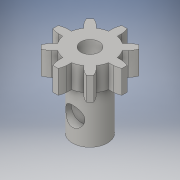
# Autodesk Inventor part: Small Gear
Saved by Autodesk Inventor 2016 (Build 200138000, 138)
## iProperties
Created: 2016-04-12
Part Number: Small Gear
Material: Generic
Document SubType Name: Modeling
Designer: rmarkowi
Density: 1 g/cm^3
Appearance: Default
Author: rmarkowi
Autodesk Inventor part; units mm, degrees
ref_plane "YZ Plane" through (0, 0, 0) normal (1, 0, 0) x (0, 1, 0)
sketch "Sketch1" plane through (0, 0, 0) normal (0, 1, 0) x (-1, 0, 0)
  line L0 (-7.4806, -1.1906) -> (-6.2374, -1.1906)
  arc A0 (-9.4068, -0.7091) -> (-7.4806, -1.1906) centre (-6.9988, 4.8297) ccw
  line L1 (-9.4068, 0) -> (-9.4068, -0.7091)
  line L2 (-9.4068, 0) -> (-9.4068, 0.7091)
  line L3 (-7.4806, 1.1906) -> (-6.2374, 1.1906)
  arc A1 (-7.4806, 1.1906) -> (-9.4068, 0.7091) centre (-6.9988, -4.8297) ccw
  line L4 (-7.4806, -1.1906) -> (-6.2374, -1.1906)
  arc A2 (-9.4068, -0.7091) -> (-7.4806, -1.1906) centre (-6.9988, 4.8297) ccw
  line L5 (-9.4068, 0) -> (-9.4068, -0.7091)
  line L6 (-9.4068, 0) -> (-9.4068, 0.7091)
  line L7 (-7.4806, 1.1906) -> (-6.2374, 1.1906)
  arc A3 (-7.4806, 1.1906) -> (-9.4068, 0.7091) centre (-6.9988, -4.8297) ccw
  line L8 (-4.4477, -6.1315) -> (-3.5686, -5.2524)
  line L9 (-4.4477, -6.1315) -> (-3.5686, -5.2524)
  line L10 (-6.6516, -6.6516) -> (-6.1502, -7.153)
  line L11 (-6.6516, -6.6516) -> (-6.1502, -7.153)
  line L12 (-6.6516, -6.6516) -> (-7.153, -6.1502)
  line L13 (-6.6516, -6.6516) -> (-7.153, -6.1502)
  line L14 (-6.1315, -4.4477) -> (-5.2524, -3.5686)
  line L15 (-6.1315, -4.4477) -> (-5.2524, -3.5686)
  arc A4 (-6.1315, -4.4477) -> (-7.153, -6.1502) centre (-1.5338, -8.364) ccw
  arc A5 (-6.1315, -4.4477) -> (-7.153, -6.1502) centre (-1.5338, -8.364) ccw
  arc A6 (-6.1502, -7.153) -> (-4.4477, -6.1315) centre (-8.364, -1.5338) ccw
  arc A7 (-6.1502, -7.153) -> (-4.4477, -6.1315) centre (-8.364, -1.5338) ccw
  line L16 (1.1906, -7.4806) -> (1.1906, -6.2374)
  line L17 (1.1906, -7.4806) -> (1.1906, -6.2374)
  line L18 (0, -9.4068) -> (0.7091, -9.4068)
  line L19 (0, -9.4068) -> (0.7091, -9.4068)
  line L20 (0, -9.4068) -> (-0.7091, -9.4068)
  line L21 (0, -9.4068) -> (-0.7091, -9.4068)
  line L22 (-1.1906, -7.4806) -> (-1.1906, -6.2374)
  line L23 (-1.1906, -7.4806) -> (-1.1906, -6.2374)
  arc A8 (-1.1906, -7.4806) -> (-0.7091, -9.4068) centre (4.8297, -6.9988) ccw
  arc A9 (-1.1906, -7.4806) -> (-0.7091, -9.4068) centre (4.8297, -6.9988) ccw
  arc A10 (0.7091, -9.4068) -> (1.1906, -7.4806) centre (-4.8297, -6.9988) ccw
  arc A11 (0.7091, -9.4068) -> (1.1906, -7.4806) centre (-4.8297, -6.9988) ccw
  line L24 (6.1315, -4.4477) -> (5.2524, -3.5686)
  line L25 (6.1315, -4.4477) -> (5.2524, -3.5686)
  line L26 (6.6516, -6.6516) -> (7.153, -6.1502)
  line L27 (6.6516, -6.6516) -> (7.153, -6.1502)
  line L28 (6.6516, -6.6516) -> (6.1502, -7.153)
  line L29 (6.6516, -6.6516) -> (6.1502, -7.153)
  line L30 (4.4477, -6.1315) -> (3.5686, -5.2524)
  line L31 (4.4477, -6.1315) -> (3.5686, -5.2524)
  arc A12 (4.4477, -6.1315) -> (6.1502, -7.153) centre (8.364, -1.5338) ccw
  arc A13 (4.4477, -6.1315) -> (6.1502, -7.153) centre (8.364, -1.5338) ccw
  arc A14 (7.153, -6.1502) -> (6.1315, -4.4477) centre (1.5338, -8.364) ccw
  arc A15 (7.153, -6.1502) -> (6.1315, -4.4477) centre (1.5338, -8.364) ccw
  line L32 (7.4806, 1.1906) -> (6.2374, 1.1906)
  line L33 (7.4806, 1.1906) -> (6.2374, 1.1906)
  line L34 (9.4068, 0) -> (9.4068, 0.7091)
  line L35 (9.4068, 0) -> (9.4068, 0.7091)
  line L36 (9.4068, 0) -> (9.4068, -0.7091)
  line L37 (9.4068, 0) -> (9.4068, -0.7091)
  line L38 (7.4806, -1.1906) -> (6.2374, -1.1906)
  line L39 (7.4806, -1.1906) -> (6.2374, -1.1906)
  arc A16 (7.4806, -1.1906) -> (9.4068, -0.7091) centre (6.9988, 4.8297) ccw
  arc A17 (7.4806, -1.1906) -> (9.4068, -0.7091) centre (6.9988, 4.8297) ccw
  arc A18 (9.4068, 0.7091) -> (7.4806, 1.1906) centre (6.9988, -4.8297) ccw
  arc A19 (9.4068, 0.7091) -> (7.4806, 1.1906) centre (6.9988, -4.8297) ccw
  line L40 (4.4477, 6.1315) -> (3.5686, 5.2524)
  line L41 (4.4477, 6.1315) -> (3.5686, 5.2524)
  line L42 (6.6516, 6.6516) -> (6.1502, 7.153)
  line L43 (6.6516, 6.6516) -> (6.1502, 7.153)
  line L44 (6.6516, 6.6516) -> (7.153, 6.1502)
  line L45 (6.6516, 6.6516) -> (7.153, 6.1502)
  line L46 (6.1315, 4.4477) -> (5.2524, 3.5686)
  line L47 (6.1315, 4.4477) -> (5.2524, 3.5686)
  arc A20 (6.1315, 4.4477) -> (7.153, 6.1502) centre (1.5338, 8.364) ccw
  arc A21 (6.1315, 4.4477) -> (7.153, 6.1502) centre (1.5338, 8.364) ccw
  arc A22 (6.1502, 7.153) -> (4.4477, 6.1315) centre (8.364, 1.5338) ccw
  arc A23 (6.1502, 7.153) -> (4.4477, 6.1315) centre (8.364, 1.5338) ccw
  line L48 (-1.1906, 7.4806) -> (-1.1906, 6.2374)
  line L49 (-1.1906, 7.4806) -> (-1.1906, 6.2374)
  line L50 (0, 9.4068) -> (-0.7091, 9.4068)
  line L51 (0, 9.4068) -> (-0.7091, 9.4068)
  line L52 (0, 9.4068) -> (0.7091, 9.4068)
  line L53 (0, 9.4068) -> (0.7091, 9.4068)
  line L54 (1.1906, 7.4806) -> (1.1906, 6.2374)
  line L55 (1.1906, 7.4806) -> (1.1906, 6.2374)
  arc A24 (1.1906, 7.4806) -> (0.7091, 9.4068) centre (-4.8297, 6.9988) ccw
  arc A25 (1.1906, 7.4806) -> (0.7091, 9.4068) centre (-4.8297, 6.9988) ccw
  arc A26 (-0.7091, 9.4068) -> (-1.1906, 7.4806) centre (4.8297, 6.9988) ccw
  arc A27 (-0.7091, 9.4068) -> (-1.1906, 7.4806) centre (4.8297, 6.9988) ccw
  line L56 (-6.1315, 4.4477) -> (-5.2524, 3.5686)
  line L57 (-6.1315, 4.4477) -> (-5.2524, 3.5686)
  line L58 (-6.6516, 6.6516) -> (-7.153, 6.1502)
  line L59 (-6.6516, 6.6516) -> (-7.153, 6.1502)
  line L60 (-6.6516, 6.6516) -> (-6.1502, 7.153)
  line L61 (-6.6516, 6.6516) -> (-6.1502, 7.153)
  line L62 (-4.4477, 6.1315) -> (-3.5686, 5.2524)
  line L63 (-4.4477, 6.1315) -> (-3.5686, 5.2524)
  arc A28 (-4.4477, 6.1315) -> (-6.1502, 7.153) centre (-8.364, 1.5338) ccw
  arc A29 (-4.4477, 6.1315) -> (-6.1502, 7.153) centre (-8.364, 1.5338) ccw
  arc A30 (-7.153, 6.1502) -> (-6.1315, 4.4477) centre (-1.5338, 8.364) ccw
  arc A31 (-7.153, 6.1502) -> (-6.1315, 4.4477) centre (-1.5338, 8.364) ccw
  arc A32 (1.1906, -6.2374) -> (3.5686, -5.2524) centre (0, 0) ccw
  arc A33 (-3.5686, -5.2524) -> (-1.1906, -6.2374) centre (0, 0) ccw
  arc A34 (-6.2374, -1.1906) -> (-5.2524, -3.5686) centre (0, 0) ccw
  arc A35 (-5.2524, 3.5686) -> (-6.2374, 1.1906) centre (0, 0) ccw
  arc A36 (-1.1906, 6.2374) -> (-3.5686, 5.2524) centre (0, 0) ccw
  arc A37 (3.5686, 5.2524) -> (1.1906, 6.2374) centre (0, 0) ccw
  arc A38 (5.2524, -3.5686) -> (6.2374, -1.1906) centre (0, 0) ccw
  arc A39 (6.2374, 1.1906) -> (5.2524, 3.5686) centre (0, 0) ccw
  point P0 (-6.907, -0.3718)
  point P1 (-6.907, 0.3718)
  point P2 (-6.907, -0.3718)
  point P3 (-6.907, 0.3718)
  point P4 (-4.6211, -5.1469)
  point P5 (-4.6211, -5.1469)
  point P6 (-5.1469, -4.6211)
  point P7 (-5.1469, -4.6211)
  point P8 (0.3718, -6.907)
  point P9 (0.3718, -6.907)
  point P10 (-0.3718, -6.907)
  point P11 (-0.3718, -6.907)
  point P12 (5.1469, -4.6211)
  point P13 (5.1469, -4.6211)
  point P14 (4.6211, -5.1469)
  point P15 (4.6211, -5.1469)
  point P16 (6.907, 0.3718)
  point P17 (6.907, 0.3718)
  point P18 (6.907, -0.3718)
  point P19 (6.907, -0.3718)
  point P20 (4.6211, 5.1469)
  point P21 (4.6211, 5.1469)
  point P22 (5.1469, 4.6211)
  point P23 (5.1469, 4.6211)
  point P24 (-0.3718, 6.907)
  point P25 (-0.3718, 6.907)
  point P26 (0.3718, 6.907)
  point P27 (0.3718, 6.907)
  point P28 (-5.1469, 4.6211)
  point P29 (-5.1469, 4.6211)
  point P30 (-4.6211, 5.1469)
  point P31 (-4.6211, 5.1469)
  dimension "d5" = 360
  constraints: 128 end point, 80 point on circle, 40 centre point, 257 other
extrude "Extrusion1" add sketch "Sketch1" along normal blind 6.35
sketch "Sketch2" plane through (0, 0, 0) normal (0, -1, 0) x (1, 0, 0)
  circle A0 centre (0, 0) radius 4.7625
  dimension "d9" = 9.525
  constraints: 1 centre point, 1 coincident
  measures "d9" diameter of A0
extrude "Extrusion2" add sketch "Sketch2" along normal blind 13.97
sketch "Sketch3" plane through (0, 6.35, 0) normal (0, 1, 0) x (1, 0, 0)
  circle A0 centre (0, 0) radius 2.5
  dimension "d12" = 5
  constraints: 1 centre point, 1 coincident
  measures "d12" diameter of A0
extrude "Extrusion3" cut sketch "Sketch3" along normal through all both and the other way through all
ref_plane "Work Plane1" through (0, 0, 2.5019) normal (0, 0, 1) x (1, 0, 0)
ref_plane "Work Plane2" through (0, 0, 4.7625) normal (0, 0, 1) x (1, 0, 0)
sketch "Sketch5" plane through (0, 0, 2.5019) normal (0, 0, 1) x (1, 0, 0)
  line L0 (2.5, -13.97) -> (-2.5, -13.97) construction
  line L1 (0.7091, 6.35) -> (-0.7091, 6.35) construction
  line L2 (0, -13.97) -> (0, -7.62) construction
  circle A0 centre (0, -7.62) radius 2.55
  point P0 (0, 0)
  dimension "d17" = 6.35
  dimension "d18" = 5.1
  constraints: 2 end point, 1 centre point, 1 coincident, 1 midpoint, 1 vertical
  measures "d17" distance of L2.start L2.end
  measures "d18" diameter of A0
sketch "Sketch6" plane through (0, 0, 4.7625) normal (0, 0, 1) x (1, 0, 0)
  line L0 (2.5, -13.97) -> (-2.5, -13.97) construction
  line L1 (0, -13.97) -> (0, -7.62) construction
  circle A0 centre (0, -7.62) radius 2.65
  point P0 (0, 0)
  dimension "d19" = 6.35
  dimension "d20" = 5.3
  constraints: 2 end point, 1 centre point, 1 coincident, 1 midpoint, 1 vertical
  measures "d19" distance of L1.start L1.end
  measures "d20" diameter of A0
loft "Loft1" cut profiles "Sketch5", "Sketch6"
body "Solid1"
